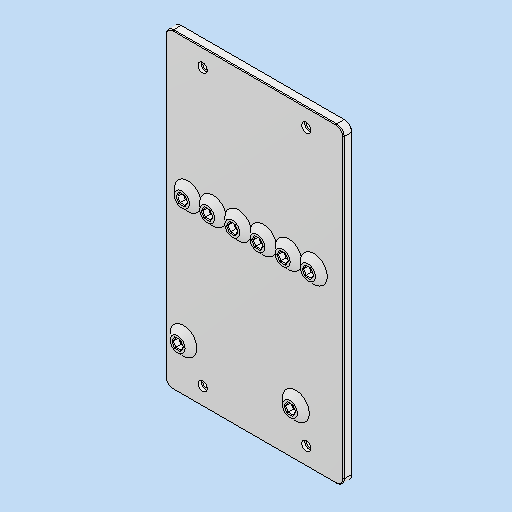
# Autodesk Inventor part: tc-bottom-tray
Saved by Autodesk Inventor 2026 (Build 300175050, 175E)
## iProperties
Created: 2025-06-05
Part Number: tc-bottom-tray
Material: ABS Plastic
Document SubType Name: Modeling
Designer: queezz
Density: 1.06 g/cm^3
Appearance: Smooth - White
Author: queezz
Autodesk Inventor part; units mm, degrees
ref_plane "XZ Plane" through (0, 0, 0) normal (0, 1, 0) x (-1, 0, 0)
ref_plane "XY Plane" through (0, 0, 0) normal (0, 0, 1) x (1, 0, 0)
sketch "Sketch1" plane through (0, 0, 0) normal (0, 0, 1) x (1, 0, 0)
  line L0 (-60, 105) -> (60, 105)
  line L1 (60, 105) -> (60, -105)
  line L2 (60, -105) -> (-60, -105)
  line L3 (-60, -105) -> (-60, 105)
  point P0 (0, 0)
  point P1 (60, 0)
  point P2 (0, 105)
  dimension "d0" = 120
  dimension "d1" = 210
  constraints: 8 end point, 2 midpoint, 2 parallel, 1 horizontal, 1 horizontal alignment, 1 perpendicular, 1 vertical alignment
  measures "d0" distance of L0.start L0.end
  measures "d1" distance of L0.end L1.end
extrude "Extrusion1" add sketch "Sketch1" along normal blind 6
fillet "Fillet1" radius 5 4 edges at (-60, 105, 3) (60, 105, 3) (60, -105, 3) (-60, -105, 3)
chamfer "Chamfer2" distance 0.5 angle 45 16 edges at (0, 105, 6) (-58.5355, 103.5355, 6) (-60, 0, 6) (-58.5355, -103.5355, 6) (0, -105, 6) (58.5355, -103.5355, 6) (60, 0, 6) (58.5355, 103.5355, 6) (0, 105, 0) (-58.5355, 103.5355, 0) (-60, 0, 0) (-58.5355, -103.5355, 0) (0, -105, 0) (58.5355, -103.5355, 0) (60, 0, 0) (58.5355, 103.5355, 0)
sketch "Sketch4" plane through (0, 0, 6) normal (0, 0, 1) x (1, 0, 0)
  line L0 (-35, -93) -> (35, -93) construction
  line L1 (-55, -105) -> (55, -105) projected
  line L2 (-35, 93) -> (35, 93) construction
  line L3 (55, 105) -> (-55, 105) projected
  point P0 (0, 0)
  point P1 (0, -93)
  point P2 (0, 93)
  dimension "d20" = 12
  dimension "d21" = 70
  dimension "d30" = 12
  constraints: 4 coincident, 4 end point, 2 horizontal, 2 midpoint, 2 vertical alignment, 1 parallel
  measures "d20" distance between parallel lines of L1 L0
  measures "d21" distance of L0.start L0.end
  measures "d30" distance between parallel lines of L3 L2
hole "Hole1" at (-35, -93, 6) at (35, -93, 6) at (-35, 93, 6) at (35, 93, 6) direction (0, 0, -1) diameter 3.6 end through all counterbore diameter 6.2 counterbore depth 2
sketch "Sketch5" plane through (0, 0, 0) normal (0, 0, -1) x (-1, 0, 0)
  line L0 (55, 105) -> (-55, 105) projected
  point P0 (45, 13)
  point P1 (0, 0)
  dimension "d45" = 92
  dimension "d46" = 45
  measures "d45" distance from line of L0 point (45, 13)
  measures "d46" horizontal distance of point (0, 0) point (45, 13)
hole "Hole2" at (-45, 13, 0) direction (0, 0, 1) diameter 3.6 end through all
sketch "Sketch7" plane through (0, 0, 6) normal (0, 0, 1) x (1, 0, 0)
  circle A0 centre (-45, 13) radius 1.8 projected
  circle A1 centre (-45, 13) radius 5
  line L0 (-46.6743, 10.1) -> (-48.3486, 13)
  line L1 (-48.3486, 13) -> (-46.6743, 15.9)
  line L2 (-46.6743, 15.9) -> (-43.3257, 15.9)
  line L3 (-43.3257, 15.9) -> (-41.6514, 13)
  line L4 (-41.6514, 13) -> (-43.3257, 10.1)
  line L5 (-43.3257, 10.1) -> (-46.6743, 10.1)
  point P0 (0, 0)
  dimension "d47" = 5.8
  dimension "d48" = 10
  constraints: 12 end point, 2 coincident, 1 centre point, 1 horizontal, 13 other
  measures "d47" distance between parallel lines of L2 L5
  measures "d48" diameter of A1
extrude "Extrusion4" add sketch "Sketch7" along normal blind 4 contours A1
chamfer "Chamfer3" distance 4 angle 45 1 edges at (-50, 13, 6)
pattern_linear "Rectangular Pattern1" count 6 spacing 17 along (1, 0, 0) of "Hole2", "Extrusion4", "Chamfer3"
sketch "Sketch6" plane through (0, 0, 0) normal (0, 0, -1) x (-1, 0, 0)
  line L0 (-27.9, -73) -> (47.9, -73) construction
  line L1 (-55, -105) -> (55, -105) projected
  point P0 (0, 0)
  point P1 (10, -73)
  dimension "d43" = 75.8
  dimension "d44" = 32
  dimension "d74" = 10
  constraints: 2 coincident, 2 end point, 1 horizontal, 1 midpoint
  measures "d43" distance of L0.start L0.end
  measures "d44" distance between parallel lines of L1 L0
  measures "d74" horizontal distance of point (0, 0) point (10, -73)
hole "Hole3" at (-47.9, -73, 0) at (27.9, -73, 0) direction (0, 0, 1) diameter 3.6 end through all
sketch "Sketch8" plane through (0, 0, 6) normal (0, 0, 1) x (1, 0, 0)
  circle A0 centre (-47.9, -73) radius 1.8 projected
  circle A1 centre (-47.9, -73) radius 5
  line L0 (-46.2257, -70.1) -> (-44.5514, -73)
  line L1 (-44.5514, -73) -> (-46.2257, -75.9)
  line L2 (-46.2257, -75.9) -> (-49.5743, -75.9)
  line L3 (-49.5743, -75.9) -> (-51.2486, -73)
  line L4 (-51.2486, -73) -> (-49.5743, -70.1)
  line L5 (-49.5743, -70.1) -> (-46.2257, -70.1)
  point P0 (0, 0)
  dimension "d64" = 5.8
  dimension "d65" = 10
  constraints: 12 end point, 2 coincident, 1 centre point, 1 horizontal, 13 other
  measures "d64" distance between parallel lines of L2 L5
  measures "d65" diameter of A1
extrude "Extrusion5" add sketch "Sketch8" along normal blind 4 contours A1
chamfer "Chamfer4" distance 4 angle 45 1 edges at (-52.9, -73, 6)
ref_plane "Work Plane1" through (-10, 0, 0) normal (1, 0, 0) x (0, 1, 0)
mirror "Mirror2" about plane through (-10, 0, 0) normal (1, 0, 0) of "Extrusion5", "Chamfer4"
chamfer "Chamfer5" distance 0.5 angle 45 56 edges at (-47.9, -70.1, 10) (-50.4115, -71.55, 10) (-50.4115, -74.45, 10) (-47.9, -75.9, 10) (-45.3885, -74.45, 10) (-45.3885, -71.55, 10) (-47.9, -74.8, 6) (27.9, -70.1, 10) (25.3885, -71.55, 10) (25.3885, -74.45, 10) (27.9, -75.9, 10) (30.4115, -74.45, 10) (30.4115, -71.55, 10) (27.9, -74.8, 6) (40, 15.9, 10) (37.4885, 14.45, 10) (37.4885, 11.55, 10) (40, 10.1, 10) (42.5115, 11.55, 10) (42.5115, 14.45, 10) (40, 11.2, 6) (23, 15.9, 10) (20.4885, 14.45, 10) (20.4885, 11.55, 10) (23, 10.1, 10) (25.5115, 11.55, 10) (25.5115, 14.45, 10) (23, 11.2, 6) (6, 15.9, 10) (8.5115, 14.45, 10) (8.5115, 11.55, 10) (6, 10.1, 10) (3.4885, 11.55, 10) (3.4885, 14.45, 10) (6, 11.2, 6) (-11, 15.9, 10) (-13.5115, 14.45, 10) (-13.5115, 11.55, 10) (-11, 10.1, 10) (-8.4885, 11.55, 10) (-8.4885, 14.45, 10) (-11, 11.2, 6) (-28, 15.9, 10) (-30.5115, 14.45, 10) (-30.5115, 11.55, 10) (-28, 10.1, 10) (-25.4885, 11.55, 10) (-25.4885, 14.45, 10) (-28, 11.2, 6) (-45, 15.9, 10) (-47.5115, 14.45, 10) (-47.5115, 11.55, 10) (-45, 10.1, 10) (-42.4885, 11.55, 10) (-42.4885, 14.45, 10) (-45, 11.2, 6)
equation "\"d0\" = width"
equation "\"d1\" = hight"
equation "\"d45\" = dindistance"
equation "\"d44\" = wago"
equation "\"d74\" = wagodelta"
equation "\"hight\" = 210"
equation "\"width\" = 120"
equation "\"dindistance\" = 92"
equation "\"wago\" = 32"
equation "\"wagodelta\" = 10"
body "Solid1"
